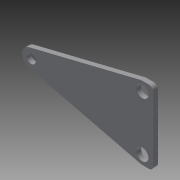
# Autodesk Inventor part: pully mount
Saved by Autodesk Inventor 2013 (Build 170138000, 138)
## iProperties
Created: 2013-09-17
Part Number: pully mount
Material: Generic
Document SubType Name: Modeling
Designer: Ian
Density: 1 g/cm^3
Mass: 8.87223 g
Surface Area: 65.8928 cm^2
Volume: 8.87223 cm^3
Author: Ian
Autodesk Inventor part; units mm, degrees
ref_plane "YZ Plane" through (0, 0, 0) normal (1, 0, 0) x (0, 1, 0)
ref_plane "XZ Plane" through (0, 0, 0) normal (0, 1, 0) x (-1, 0, 0)
ref_plane "XY Plane" through (0, 0, 0) normal (0, 0, 1) x (1, 0, 0)
sketch "Sketch1" plane through (0, 0, 0) normal (0, 0, 1) x (1, 0, 0)
  line L0 (7.62, 0) -> (12.065, 0)
  line L1 (15.24, 3.175) -> (15.24, 47.625)
  line L2 (12.065, 50.8) -> (7.62, 50.8)
  circle A0 centre (7.62, 44.45) radius 4.1656
  circle A1 centre (7.62, 6.35) radius 4.1656
  arc A2 (15.24, 47.625) -> (12.065, 50.8) centre (12.065, 47.625) ccw
  arc A3 (12.065, 0) -> (15.24, 3.175) centre (12.065, 3.175) ccw
  circle A4 centre (-69.85, 25.4) radius 3.175
  arc A5 (-71.3663, 31.5663) -> (-71.3663, 19.2337) centre (-69.85, 25.4) ccw
  arc A6 (7.62, 50.8) -> (6.1037, 50.6163) centre (7.62, 44.45) ccw
  arc A7 (6.1037, 0.1837) -> (7.62, 0) centre (7.62, 6.35) ccw
  line L3 (-69.85, 25.4) -> (7.62, 44.45) construction
  line L4 (-69.85, 25.4) -> (7.62, 6.35) construction
  line L5 (15.24, 25.4) -> (-69.85, 25.4) construction
  line L6 (-71.3663, 31.5663) -> (6.1037, 50.6163)
  line L7 (-71.3663, 19.2337) -> (6.1037, 0.1837)
  line L8 (0, 42.5762) -> (0, 0) construction
  point P0 (15.24, 50.8)
  point P1 (15.24, 0)
  dimension "d1" = 50.8
  dimension "d2" = 38.1
  dimension "d3" = 6.35
  dimension "d4" = 8.3312
  dimension "d5" = 8.3312
  dimension "d9" = 3.175
  dimension "d12" = 6.35
  dimension "d14" = 12.7
  dimension "d16" = 15.24
  dimension "d18" = 76.185
  dimension "d19" = 50.8
  dimension "d20" = 25.4
  dimension "d21" = 85.09
  dimension "d22" = 69.85
  dimension "d23" = 76.185
  dimension "d24" = 27.63
  dimension "d25" = 27.63
  dimension "d26" = 152.37
  dimension "d27" = 13.815
  dimension "d28" = 4.445
  dimension "d29" = 77.47
  dimension "d30" = 19.05
  dimension "d31" = 13.815
  dimension "d32" = 13.815
  dimension "d33" = 7.62
  dimension "d34" = 6.35
  dimension "d35" = 90
  dimension "d36" = 7.62
  dimension "d37" = 6.35
  dimension "d38" = 4.445
  dimension "d39" = 3.175
  constraints: 18 end point, 10 point on circle, 10 tangent, 8 centre point, 5 coincident, 5 point on line, 3 parallel, 1 equal radius, 1 horizontal, 1 midpoint, 1 perpendicular, 1 other
  measures "d1" distance of point (15.24, 50.8) point (15.24, 0)
  measures "d2" distance of point (7.62, 6.35) point (7.62, 44.45)
  measures "d3" distance from line of L0 point (7.62, 6.35)
  measures "d4" diameter of A0
  measures "d5" diameter of A1
  measures "d9" radius of A2
  measures "d12" diameter of A4
  measures "d14" diameter of A5
  measures "d16" distance between parallel lines of L1 L8
  measures "d18" angle of L1 L3
  measures "d19" distance from line of L8.end L2
  measures "d20" vertical distance of L8.end A4.centre
  measures "d21" distance from line of L1 A4.centre
  measures "d22" horizontal distance of L8.end A4.centre
  measures "d23" angle of L1 L7
  measures "d24" angle of L6 L7
  measures "d25" angle of L3 L4
  measures "d28" distance of L2.start L2.end
  measures "d29" horizontal distance of L6.end L6.start
  measures "d30" vertical distance of L6.end L6.start
  measures "d31" angle of L5 L4
  measures "d32" angle of L7 L5
  measures "d33" distance from line of L8 A1.centre
  measures "d34" vertical distance of L8.end A1.centre
  measures "d35" angle of L1 L5
  measures "d36" distance from line of L1 point (7.62, 44.45)
  measures "d37" distance from line of L6 A0.centre
  measures "d38" horizontal distance of L3.end A2.centre
  measures "d39" vertical distance of A0.centre A2.centre
extrude "Extrusion1" add sketch "Sketch1" along normal blind 3.175
equation "\"d5\" = d4"
body "Solid1"
